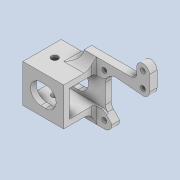
# Autodesk Inventor part: test_bridge_2
Saved by Autodesk Inventor 2020 (Build 240168000, 168)
## iProperties
Created: 2022-02-03
Part Number: test_bridge_2
Material: Generic
Document SubType Name: Modeling
Designer: Shuang Peng
Density: 1 g/cm^3
Appearance: Default
Author: Shuang Peng
Autodesk Inventor part; units mm, degrees
ref_plane "YZ Plane" through (0, 0, 0) normal (1, 0, 0) x (0, 1, 0)
ref_plane "XZ Plane" through (0, 0, 0) normal (0, 1, 0) x (-1, 0, 0)
ref_plane "XY Plane" through (0, 0, 0) normal (0, 0, 1) x (1, 0, 0)
sketch "Sketch1" plane through (0, 0, 0) normal (0, 0, 1) x (1, 0, 0)
  circle A0 centre (-0.5, 9.9) radius 0.95 projected
  circle A1 centre (-0.5, 15.9) radius 0.95 projected
  circle A2 centre (-15.7, -8.5) radius 0.95 projected
  circle A3 centre (-15.7, 8.5) radius 0.95 projected
  line L0 (21, -18) -> (18, -21) projected
  line L1 (21, -18) -> (21, 18) projected
  line L2 (18, 21) -> (21, 18) projected
  line L3 (18, 21) -> (-18, 21) projected
  line L4 (-21, 18) -> (-18, 21) projected
  line L5 (-21, 18) -> (-21, -18) projected
  line L6 (-18, -21) -> (-21, -18) projected
  line L7 (-18, -21) -> (18, -21) projected
  line L8 (-7, 9.5) -> (-11, 9.5) projected
  arc A4 (-11, 16.5) -> (-11, 9.5) centre (-11, 13) ccw projected
  line L9 (-11, 16.5) -> (-7, 16.5) projected
  arc A5 (-7, 9.5) -> (-7, 16.5) centre (-7, 13) ccw projected
  arc A6 (-7, -16.5) -> (-7, -9.5) centre (-7, -13) ccw projected
  line L10 (-7, -16.5) -> (-11, -16.5) projected
  arc A7 (-11, -9.5) -> (-11, -16.5) centre (-11, -13) ccw projected
  line L11 (-11, -9.5) -> (-7, -9.5) projected
  arc A8 (-9.7, -1.5) -> (-9.7, 1.5) centre (-9.7, 0) ccw projected
  line L12 (-9.7, -1.5) -> (-15.7, -1.5) projected
  arc A9 (-15.7, 1.5) -> (-15.7, -1.5) centre (-15.7, 0) ccw projected
  line L13 (-15.7, 1.5) -> (-9.7, 1.5) projected
  line L14 (8.5, 1) -> (8.5, 7) projected
  arc A10 (11.5, 7) -> (8.5, 7) centre (10, 7) ccw projected
  line L15 (11.5, 7) -> (11.5, 1) projected
  arc A11 (8.5, 1) -> (11.5, 1) centre (10, 1) ccw projected
  arc A12 (12, 16.15) -> (12, 17.65) centre (12, 16.9) ccw projected
  line L16 (12, 16.15) -> (8, 16.15) projected
  arc A13 (8, 17.65) -> (8, 16.15) centre (8, 16.9) ccw projected
  line L17 (8, 17.65) -> (12, 17.65) projected
  line L18 (0.95, 2) -> (0.95, -2) projected
  arc A14 (-0.55, -2) -> (0.95, -2) centre (0.2, -2) ccw projected
  line L19 (-0.55, -2) -> (-0.55, 2) projected
  arc A15 (0.95, 2) -> (-0.55, 2) centre (0.2, 2) ccw projected
  line L20 (1, -17) -> (1, -7) projected
  arc A16 (3, -5) -> (1, -7) centre (3, -7) ccw projected
  line L21 (3, -5) -> (17, -5) projected
  arc A17 (19, -7) -> (17, -5) centre (17, -7) ccw projected
  line L22 (19, -7) -> (19, -17) projected
  arc A18 (17, -19) -> (19, -17) centre (17, -17) ccw projected
  line L23 (17, -19) -> (3, -19) projected
  arc A19 (1, -17) -> (3, -19) centre (3, -17) ccw projected
  circle A20 centre (4.5, 4) radius 0.85 projected
  circle A21 centre (-12.7, -5.5) radius 0.85 projected
  circle A22 centre (-12.7, 5.5) radius 0.85 projected
  circle A23 centre (-2.8, 0) radius 0.85 projected
  circle A24 centre (15.5, 4) radius 0.85 projected
  circle A25 centre (10, 13.9) radius 0.85 projected
  line L24 (-12.7, -8.5) -> (-15.1828, -5.8668) projected
  arc A26 (-16, -3.8087) -> (-15.1828, -5.8668) centre (-13, -3.8087) ccw projected
  line L25 (-16, -3.8087) -> (-16, -2) projected
  line L26 (-16, 2) -> (-16, 3.8087) projected
  arc A27 (-15.1828, 5.8668) -> (-16, 3.8087) centre (-13, 3.8087) ccw projected
  line L27 (-15.1828, 5.8668) -> (-12.7, 8.5) projected
  arc A28 (-12.7, 8.5) -> (-18.4375, 9.7273) centre (-15.7, 8.5) ccw projected
  arc A29 (-18.4375, -9.7273) -> (-12.7, -8.5) centre (-15.7, -8.5) ccw projected
  line L28 (-15.7, 8.5) -> (-15.7, 11.5)
  line L29 (-15.7, -8.5) -> (-15.7, -11.5)
  line L30 (-16, 2) -> (-16, -2)
  line L31 (-15.7, -11.5) -> (-35.7, -11.5)
  line L32 (-35.7, -11.5) -> (-35.7, 11.5)
  line L33 (-35.7, 11.5) -> (-15.7, 11.5)
  line L34 (-15.7, 11.5) -> (-15.7, -11.5)
  point P0 (0, 0)
  dimension "d0" = 20
  dimension "d1" = 23
  constraints: 14 end point, 3 vertical, 2 parallel, 2 point on circle, 1 horizontal, 1 perpendicular
  measures "d0" distance of L32.end L33.end
  measures "d1" distance of L31.end L32.end
extrude "Extrusion1" add sketch "Sketch1" along normal blind 3 contours A2 L34 A26 L24 A29 L29 | A2 L29 L31 L5 L33 L28 A3 L34 A27 L26 L30 A9 L25 A26 | L31 L32 L33 L5 | A9 L30 | L34 A3 L28 A28 L27 A27
sketch "Sketch2" plane through (0, 0, 3) normal (0, 0, 1) x (1, 0, 0)
  circle A0 centre (-0.5, 9.9) radius 0.95 projected
  circle A1 centre (-0.5, 15.9) radius 0.95 projected
  circle A2 centre (-15.7, -8.5) radius 0.95 projected
  circle A3 centre (-15.7, 8.5) radius 0.95 projected
  line L0 (21, -18) -> (18, -21) projected
  line L1 (21, -18) -> (21, 18) projected
  line L2 (18, 21) -> (21, 18) projected
  line L3 (18, 21) -> (-18, 21) projected
  line L4 (-21, 18) -> (-18, 21) projected
  line L5 (-21, 18) -> (-21, -18) projected
  line L6 (-18, -21) -> (-21, -18) projected
  line L7 (-18, -21) -> (18, -21) projected
  line L8 (-7, 9.5) -> (-11, 9.5) projected
  arc A4 (-11, 16.5) -> (-11, 9.5) centre (-11, 13) ccw projected
  line L9 (-11, 16.5) -> (-7, 16.5) projected
  arc A5 (-7, 9.5) -> (-7, 16.5) centre (-7, 13) ccw projected
  arc A6 (-7, -16.5) -> (-7, -9.5) centre (-7, -13) ccw projected
  line L10 (-7, -16.5) -> (-11, -16.5) projected
  arc A7 (-11, -9.5) -> (-11, -16.5) centre (-11, -13) ccw projected
  line L11 (-11, -9.5) -> (-7, -9.5) projected
  arc A8 (-9.7, -1.5) -> (-9.7, 1.5) centre (-9.7, 0) ccw projected
  line L12 (-9.7, -1.5) -> (-15.7, -1.5) projected
  arc A9 (-15.7, 1.5) -> (-15.7, -1.5) centre (-15.7, 0) ccw projected
  line L13 (-15.7, 1.5) -> (-9.7, 1.5) projected
  line L14 (8.5, 1) -> (8.5, 7) projected
  arc A10 (11.5, 7) -> (8.5, 7) centre (10, 7) ccw projected
  line L15 (11.5, 7) -> (11.5, 1) projected
  arc A11 (8.5, 1) -> (11.5, 1) centre (10, 1) ccw projected
  arc A12 (12, 16.15) -> (12, 17.65) centre (12, 16.9) ccw projected
  line L16 (12, 16.15) -> (8, 16.15) projected
  arc A13 (8, 17.65) -> (8, 16.15) centre (8, 16.9) ccw projected
  line L17 (8, 17.65) -> (12, 17.65) projected
  line L18 (0.95, 2) -> (0.95, -2) projected
  arc A14 (-0.55, -2) -> (0.95, -2) centre (0.2, -2) ccw projected
  line L19 (-0.55, -2) -> (-0.55, 2) projected
  arc A15 (0.95, 2) -> (-0.55, 2) centre (0.2, 2) ccw projected
  line L20 (1, -17) -> (1, -7) projected
  arc A16 (3, -5) -> (1, -7) centre (3, -7) ccw projected
  line L21 (3, -5) -> (17, -5) projected
  arc A17 (19, -7) -> (17, -5) centre (17, -7) ccw projected
  line L22 (19, -7) -> (19, -17) projected
  arc A18 (17, -19) -> (19, -17) centre (17, -17) ccw projected
  line L23 (17, -19) -> (3, -19) projected
  arc A19 (1, -17) -> (3, -19) centre (3, -17) ccw projected
  circle A20 centre (4.5, 4) radius 0.85 projected
  circle A21 centre (-12.7, -5.5) radius 0.85 projected
  circle A22 centre (-12.7, 5.5) radius 0.85 projected
  circle A23 centre (-2.8, 0) radius 0.85 projected
  circle A24 centre (15.5, 4) radius 0.85 projected
  circle A25 centre (10, 13.9) radius 0.85 projected
  line L24 (-0.5, 9.9) -> (-0.5, 15.9) construction
  line L25 (2, 9.9) -> (2, 15.9)
  line L26 (-3, 15.9) -> (-3, 9.9)
  arc A26 (-3, 9.9) -> (2, 9.9) centre (-0.5, 9.9) ccw
  arc A27 (2, 15.9) -> (-3, 15.9) centre (-0.5, 15.9) ccw
  line L27 (-15.7, 11.5) -> (-35.7, 11.5) projected
  line L28 (-15.7, 11.5) -> (-3, 11.5)
  line L29 (-0.5, 12.9) -> (-0.5, 7.4)
  line L30 (-15.1828, 5.8668) -> (-12.7, 8.5) projected
  line L31 (-0.5, 7.4) -> (-12.7, 8.5)
  arc A28 (-12.7, 8.5) -> (-15.7, 11.5) centre (-15.7, 8.5) ccw projected
  point P0 (0, 0)
  dimension "d4" = 5
  constraints: 14 end point, 5 point on circle, 4 tangent, 2 centre point, 1 midpoint, 1 parallel, 1 perpendicular, 1 point on line, 1 vertical
  measures "d4" diameter of A27
extrude "Extrusion2" add sketch "Sketch2" against normal blind 3 contours A5 L28 L26 A26 L31 A28 A4 L8 | L8 A4 L28 A5 | L26 A27 L25 A26 L31
fillet "Fillet1" radius 4 1 edges at (-12.7, 8.5, 1.5)
fillet "Fillet2" radius 2 1 edges at (-3, 11.5, 1.5)
sketch "Sketch3" plane through (-35.7, -11.5, 0) normal (-1, 0, 0) x (0, 0, 1)
  line L0 (0, 23) -> (0, 0) projected
  line L1 (0, 0) -> (3, 0) projected
  line L2 (3, 23) -> (3, 0) projected
  line L3 (0, 23) -> (3, 23) projected
  line L4 (3, 23) -> (15, 23)
  line L5 (15, 23) -> (15, 0)
  line L6 (15, 0) -> (3, 0)
  line L7 (3, 0) -> (3, 23)
  point P0 (0, 11.5)
  dimension "d9" = 12
  dimension "d10" = 23
  constraints: 8 end point, 2 parallel, 1 horizontal, 1 perpendicular
  measures "d9" distance of L5.end L6.end
  measures "d10" distance of L4.end L5.end
extrude "Extrusion3" add sketch "Sketch3" against normal blind 16 contours L4 L5 L6 L2
sketch "Sketch4" plane through (-35.7, -11.5, 0) normal (-1, 0, 0) x (0, 0, 1)
  line L0 (0, 23) -> (0, 0) projected
  line L1 (0, 0) -> (15, 0) projected
  line L2 (15, 0) -> (15, 23) projected
  line L3 (0, 23) -> (15, 23) projected
  line L4 (0, 23) -> (15, 23) projected
  line L5 (0, 23) -> (0, 0) projected
  line L6 (15, 23) -> (0, 0)
  line L7 (0, 0) -> (15, 0) projected
  line L8 (0, 0) -> (15, 0)
  line L9 (15, 0) -> (0, 23)
  line L10 (12.75, 16.75) -> (12.75, 6.25)
  line L11 (12.75, 6.25) -> (2.25, 6.25)
  line L12 (2.25, 6.25) -> (2.25, 16.75)
  line L13 (2.25, 16.75) -> (12.75, 16.75)
  line L14 (12.75, 16.75) -> (2.25, 6.25) construction
  line L15 (12.75, 6.25) -> (2.25, 16.75) construction
  point P0 (0, 11.5)
  point P1 (7.5, 11.5)
  dimension "d13" = 10.5
  dimension "d14" = 10.5
  constraints: 18 end point, 3 equal length, 3 midpoint, 1 perpendicular, 1 vertical
  measures "d13" distance of L10.start L10.end
  measures "d14" distance of L10.end L11.end
extrude "Extrusion4" cut sketch "Sketch4" against normal blind 25 contours L13 L6 L9 | L9 L6 L11 L12 L13 | L6 L9 L11 | L13 L10 L11 L9 L6
sketch "Sketch5" plane through (-35.7, -11.5, 15) normal (0, 0, 1) x (1, 0, 0)
  line L0 (0, 0) -> (0, 23) projected
  line L1 (0, 0) -> (16, 0) projected
  line L2 (16, 23) -> (16, 0) projected
  line L3 (0, 23) -> (16, 23) projected
  arc A0 (20.5172, 17.3668) -> (20.0689, 16.75) centre (22.7, 15.3087) ccw projected
  line L4 (20.5172, 17.3668) -> (21.6665, 18.5857) projected
  arc A1 (24.936, 19.8254) -> (21.6665, 18.5857) centre (24.5768, 15.8416) ccw projected
  line L5 (24.936, 19.8254) -> (35.2, 18.9) projected
  arc A2 (35.2, 18.9) -> (37.7, 21.4) centre (35.2, 21.4) ccw projected
  line L6 (37.7, 21.4) -> (37.7, 27.4) projected
  arc A3 (37.7, 27.4) -> (32.7, 27.4) centre (35.2, 27.4) ccw projected
  line L7 (32.7, 27.4) -> (32.7, 25) projected
  arc A4 (30.7, 23) -> (32.7, 25) centre (30.7, 25) ccw projected
  line L8 (30.7, 23) -> (16, 23) projected
  line L9 (16, 23) -> (16, 16.75) projected
  line L10 (16, 16.75) -> (20.0689, 16.75) projected
  circle A5 centre (20, 20) radius 0.95 projected
  circle A6 centre (35.2, 21.4) radius 0.95 projected
  circle A7 centre (35.2, 27.4) radius 0.95 projected
  circle A8 centre (20, 3) radius 0.95 projected
  line L11 (20.0689, 6.25) -> (16, 6.25) projected
  line L12 (16, 6.25) -> (16, 0) projected
  line L13 (16, 0) -> (20, 0) projected
  arc A9 (20, 0) -> (23, 3) centre (20, 3) ccw projected
  line L14 (23, 3) -> (20.5172, 5.6332) projected
  arc A10 (20.0689, 6.25) -> (20.5172, 5.6332) centre (22.7, 7.6913) ccw projected
  line L15 (0, 23) -> (30.7, 23) projected
  line L16 (0, 23) -> (17, 23)
  line L17 (17, 23) -> (17, 19)
  line L18 (17, 19) -> (0, 19)
  line L19 (0, 19) -> (0, 23)
  line L20 (0, 0) -> (17, 0)
  line L21 (17, 0) -> (17, 4)
  line L22 (17, 4) -> (0, 4)
  line L23 (0, 4) -> (0, 0)
  point P0 (35.7, 11.5)
  point P1 (0, 4)
  dimension "d17" = 17
  dimension "d18" = 4
  dimension "d19" = 17
  dimension "d20" = 4
  constraints: 16 end point, 4 parallel, 2 horizontal, 2 perpendicular
  measures "d17" distance of L17.end L18.end
  measures "d18" distance of L16.end L17.end
  measures "d19" distance of L22.end L21.end
  measures "d20" distance of L21.end L20.end
extrude "Extrusion5" cut sketch "Sketch5" against normal blind 20 contours L0 L22 L2 L1 | L2 L22 L21 L13 | L0 L3 L2 L18 | L2 L8 L17 L18
thicken "Thicken1" operation add thickness 5 both sides no extend neighbours yes toward (-1, 0, 0) faces at (-18.7, 10.1667, 1)
thicken "Thicken2" operation add thickness 5 both sides no extend neighbours yes toward (-1, 0, 0) faces at (-18.7, -10.1667, 2)
fillet "Fillet3" radius 4 2 edges at (-23.7, -7.5, 1.5) (-23.7, 7.5, 1.5)
fillet "Fillet4" radius 4 4 edges at (-25.6999, -7.5, 3) (-21.7, -7.5, 3) (-25.6999, 7.5, 3) (-21.7, 7.5, 3)
fillet "Fillet5" radius 1 4 edges at (-19.7, 9.5, 3) (-19.7, 6.375, 3) (-19.7, -9.4999, 3) (-19.7, -6.375, 3)
fillet "Fillet6" radius 3 2 edges at (-15.6311, 5.25, 2.625) (-15.6311, -5.25, 2.625)
sketch "Sketch6" plane through (0, 0, 0) normal (0, 0, -1) x (-1, 0, 0)
  circle A0 centre (15.7, -8.5) radius 0.95 projected
  circle A1 centre (15.7, 8.5) radius 0.95 projected
  line L0 (27.7, -7.5) -> (35.7, -7.5) projected
  line L1 (35.7, 7.5) -> (35.7, -7.5) projected
  line L2 (35.7, 7.5) -> (27.7, 7.5) projected
  arc A2 (23.7, 11.5) -> (27.7, 7.5) centre (27.7, 11.5) ccw projected
  line L3 (23.7, 11.5) -> (5, 11.5) projected
  arc A3 (3, 13.5) -> (5, 11.5) centre (5, 13.5) ccw projected
  line L4 (3, 13.5) -> (3, 15.9) projected
  arc A4 (3, 15.9) -> (-2, 15.9) centre (0.5, 15.9) ccw projected
  line L5 (-2, 15.9) -> (-2, 9.9) projected
  arc A5 (-2, 9.9) -> (0.5, 7.4) centre (0.5, 9.9) ccw projected
  line L6 (0.5, 7.4) -> (10.764, 8.3254) projected
  arc A6 (14.0335, 7.0857) -> (10.764, 8.3254) centre (11.1232, 4.3416) ccw projected
  line L7 (15.1828, 5.8668) -> (14.0335, 7.0857) projected
  arc A7 (16, 3.8087) -> (15.1828, 5.8668) centre (13, 3.8087) ccw projected
  line L8 (16, -3.8087) -> (16, 3.8087) projected
  arc A8 (15.1828, -5.8668) -> (16, -3.8087) centre (13, -3.8087) ccw projected
  line L9 (12.7, -8.5) -> (15.1828, -5.8668) projected
  arc A9 (12.7, -8.5) -> (15.7, -11.5) centre (15.7, -8.5) ccw projected
  line L10 (23.7, -11.5) -> (15.7, -11.5) projected
  arc A10 (27.7, -7.5) -> (23.7, -11.5) centre (27.7, -11.5) ccw projected
  circle A11 centre (0.5, 9.9) radius 0.95 projected
  circle A12 centre (0.5, 15.9) radius 0.95 projected
  line L11 (35.7, -5.25) -> (35.7, 5.25) projected
  line L12 (35.7, 0) -> (27.7, 0)
  line L13 (26.7, 0) -> (28.7, 0) construction
  line L14 (26.7, -4) -> (28.7, -4)
  line L15 (28.7, 4) -> (26.7, 4)
  arc A13 (26.7, 4) -> (26.7, -4) centre (26.7, 0) ccw
  arc A14 (28.7, -4) -> (28.7, 4) centre (28.7, 0) ccw
  point P0 (0, 0)
  dimension "d31" = 8
  dimension "d32" = 1
  dimension "d33" = 8
  constraints: 10 end point, 4 point on circle, 4 tangent, 2 centre point, 2 midpoint, 1 parallel, 1 perpendicular, 1 point on line
  measures "d31" distance of L12.start L12.end
  measures "d32" distance of L12.end L13.end
  measures "d33" diameter of A14
extrude "Extrusion6" cut sketch "Sketch6" against normal blind 25 contours A13 L15 A14 L14
sketch "Sketch7" plane through (-35.7, -7.5, 15) normal (0, -1, 0) x (1, 0, 0)
  line L0 (8, -8) -> (8, -15) projected
  line L1 (16, -8) -> (8, -8) projected
  line L2 (16, 0) -> (16, -8) projected
  line L3 (0, 0) -> (16, 0) projected
  line L4 (0, -15) -> (0, 0) projected
  line L5 (8, -15) -> (0, -15) projected
  line L6 (0, -12.75) -> (0, -2.25) projected
  line L7 (0, -7.5) -> (5, -7.5)
  circle A0 centre (5, -7.5) radius 1.3
  point P0 (35.7, -15)
  dimension "d36" = 5
  dimension "d37" = 2.6
  constraints: 2 end point, 1 centre point, 1 coincident, 1 horizontal, 1 midpoint
  measures "d36" distance of L7.start L7.end
  measures "d37" diameter of A0
extrude "Extrusion7" cut sketch "Sketch7" against normal blind 25 contours A0
body "Solid1"
